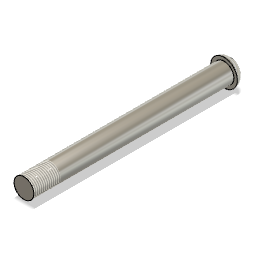
HandlePin v2 (Autodesk Fusion 360 design; units mm, degrees)
Autodesk Fusion 360 part; units mm, degrees
sketch "Sketch1" plane through (0, 0, 0) normal (0, 0, 1) x (1, 0, 0)
  circle A0 centre (74.2368, 105.6989) radius 7.5
  dimension "d13" = 15
  measures "d13" diameter of A0
extrude "Extrude1" add sketch "Sketch1" along normal blind 150
sketch "Sketch2" plane through (0, 0, 0) normal (0, 0, -1) x (-1, 0, 0)
  circle A0 centre (-74.2368, 105.6989) radius 7.5
  circle A1 centre (-74.2368, 105.6989) radius 10
  dimension "d16" = 20
  constraint horizontal A0.centre A1.centre
  constraint concentric A0 A1
  measures "d16" diameter of A1
extrude "Extrude2" add sketch "Sketch2" along normal blind 6 draft 6 contours A0 | A1
fillet "Fillet1" radius 6 1 edges at (84.148, 109.5431, -6)
sketch "Sketch3" plane through (0, 0, -6) normal (0, 0, -1) x (-1, 0, 0)
  circle A0 centre (-74.2368, 105.6989) radius 4
  line L0 (-75.2368, 112.1989) -> (-73.2368, 112.1989)
  line L1 (-73.2368, 112.1989) -> (-73.2368, 99.1989)
  line L2 (-73.2368, 99.1989) -> (-75.2368, 99.1989)
  line L3 (-75.2368, 99.1989) -> (-75.2368, 112.1989)
  dimension "d20" = 2
  dimension "d21" = 1
  dimension "d22" = 6.5
  constraint horizontal L0
  constraint vertical L1
  constraint horizontal L2
  constraint vertical L3
  measures "d20" distance of L0.start L0.end
  measures "d21" distance of A0.centre L1
  measures "d22" distance of A0.centre L2
extrude "Extrude3" cut sketch "Sketch3" against normal blind 2 contours A0 L1 L3 | A0 L0 L1 L3 | A0 L1 L2 L3
thread "Thread1" "ISO Metric profile 15.0 M15x1.5 6g" major diameter 14.85 minor diameter 13.1369 pitch 1.5 angle 60 resizes the face on face at (81.7275, 105.325, 100) from (74.2368, 105.6989, 130) to (74.2368, 105.6989, 150)
